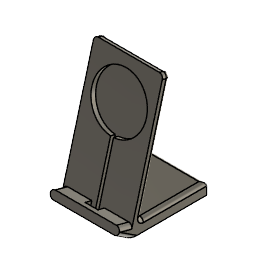
Phone stand (Autodesk Fusion 360 design; units mm, degrees)
part number: 2026-01-15-00-13-54-306
Autodesk Fusion 360 part; units mm, degrees
sketch "Sketch1" plane through (0, 0, 0) normal (1, 0, 0) x (0, 1, 0)
  line L0 (0, 0) -> (70, 0)
  line L1 (70, 0) -> (70, 12)
  line L2 (70, 12) -> (3.2154, 12)
  line L3 (25.9915, 127.9111) -> (33.7189, 125.8405)
  line L4 (33.7189, 125.8405) -> (0.59, 2.202)
  line L5 (0.59, 2.202) -> (-7.1374, 4.2726)
  line L6 (-7.1374, 4.2726) -> (25.9915, 127.9111)
  line L7 (-7.1374, 4.2726) -> (-19.6944, 7.6372)
  line L8 (-19.6944, 7.6372) -> (-17.6239, 15.3646)
  line L9 (-17.6239, 15.3646) -> (-5.0668, 12)
  line L10 (0, 0) -> (3.2154, 12)
  line L11 (-19.6944, 7.6372) -> (-8, 0)
  line L12 (-8, 0) -> (0, 0)
  dimension "d1" = 12
  dimension "d3" = 128
  dimension "d4" = 8
  dimension "d5" = 13
  dimension "d6" = 8
  dimension "d7" = 75
  dimension "d8" = 70
  dimension "d10" = 12
  dimension "d11" = 8
  constraint horizontal L0
  constraint vertical L1
  constraint horizontal L2
  constraint coincident L0.start L10.start
  constraint perpendicular L6 L7
  constraint perpendicular L7 L8
  constraint coincident L6 L9.end
  constraint perpendicular L6 L9
  constraint parallel L4 L10
  constraint coincident L4 L2.end
  constraint perpendicular L4 L5
  constraint perpendicular L1 L12
  measures "d1" distance of L0 L2
  measures "d3" distance of L3 L5
  measures "d4" distance of L4 L6
  measures "d5" distance of L6 L8
  measures "d6" distance of L7 L9
  measures "d7" angle of L2 L4
  measures "d8" distance of L0.start L1
  measures "d10" distance of L9.end L12
  measures "d11" distance of L0.start L11.end
extrude "Extrude1" add sketch "Sketch1" along normal blind 70
sketch "Sketch2" plane through (0, -7.7274, 2.0706) normal (0, -0.965926, 0.258819) x (1, 0, 0)
  line L0 (0, 130.2797) -> (0, 10.2797)
  line L1 (0, 10.2797) -> (70, 10.2797)
  line L2 (70, 10.2797) -> (70, 130.2797)
  line L3 (70, 130.2797) -> (0, 130.2797)
  circle A0 centre (35, 92.2797) radius 27.75
  line L4 (33.5, 10.2797) -> (36.5, 10.2797)
  line L5 (36.5, 10.2797) -> (36.5, 64.5703)
  line L6 (33.5, 64.5703) -> (33.5, 10.2797)
  dimension "d14" = 55.5
  dimension "d15" = 82
  dimension "d16" = 35
  dimension "d17" = 3
  constraint horizontal L4
  constraint vertical L5
  constraint vertical L6
  constraint coincident L1 L4.start
  constraint coincident A0 L6.start
  constraint coincident A0 L5.end
  constraint midpoint L1 L4
  measures "d14" diameter of A0
  measures "d15" distance of L1 A0.centre
  measures "d16" distance of L2 A0.centre
  measures "d17" distance of L5 L6
extrude "Extrude2" cut sketch "Sketch2" against normal blind 5 contours L1 A0 L4 L5 L6 | A0
sketch "Sketch3" plane through (0, 2.6606, 9.9294) normal (0, 0.258819, 0.965926) x (-1, 0, 0)
  line L0 (0, 8) -> (0, 21)
  line L1 (0, 21) -> (-70, 21)
  line L2 (-70, 21) -> (-70, 8)
  line L3 (-70, 8) -> (-36.5, 8)
  line L4 (-36.5, 8) -> (-36.5, 3)
  line L5 (-36.5, 3) -> (-33.5, 3)
  line L6 (-33.5, 3) -> (-33.5, 8)
  line L7 (-33.5, 8) -> (0, 8)
  line L8 (-28.5, 8) -> (-41.5, 8)
  line L9 (-41.5, 8) -> (-41.5, 15)
  line L10 (-41.5, 15) -> (-28.5, 15)
  line L11 (-28.5, 15) -> (-28.5, 8)
  line L12 (-33.5, 3) -> (-36.5, 3)
  line L13 (-36.5, 3) -> (-36.5, 8)
  line L14 (-36.5, 8) -> (-33.5, 8)
  line L15 (-33.5, 8) -> (-33.5, 3)
  dimension "d20" = 13
  dimension "d21" = 7
  constraint horizontal L8
  constraint vertical L9
  constraint horizontal L10
  constraint vertical L11
  constraint collinear L3 L8
  constraint horizontal L12
  constraint vertical L13
  constraint horizontal L14
  constraint vertical L15
  constraint coincident L3.end L4.start
  constraint coincident L5.end L6.start
  constraint midpoint L8 L14
  measures "d20" distance of L9 L11
  measures "d21" distance of L8 L10
extrude "Extrude3" cut sketch "Sketch3" against normal blind 13 contours L3 L7 L8 L9 L10 L11 L14 | L4 L5 L6 L8 L12 L13 L14 L15
sketch "Sketch4" plane through (0, 0, 0) normal (0, 0, -1) x (1, 0, 0)
  line L0 (33.5, 3.1058) -> (33.5, 8)
  line L1 (33.5, 8) -> (0, 8)
  line L2 (0, 8) -> (0, -70)
  line L3 (0, -70) -> (70, -70)
  line L4 (70, -70) -> (70, 8)
  line L5 (70, 8) -> (36.5, 8)
  line L6 (36.5, 8) -> (36.5, 3.1058)
  line L7 (36.5, 3.1058) -> (33.5, 3.1058)
  line L8 (33.5, 3.1058) -> (36.5, 3.1058)
  line L9 (36.5, 3.1058) -> (36.5, -70)
  line L10 (36.5, -70) -> (33.5, -70)
  line L11 (33.5, -70) -> (33.5, 3.1058)
  circle A0 centre (35, -31) radius 25
  dimension "d24" = 3
  dimension "d25" = 39
  dimension "d26" = 35
  dimension "d27" = 50
  constraint horizontal L8
  constraint vertical L9
  constraint horizontal L10
  constraint vertical L11
  constraint coincident L3 L9.end
  constraint coincident L0.start L7.end
  measures "d24" distance of L9 L11
  measures "d25" distance of L3 A0.centre
  measures "d26" distance of L4 A0.centre
  measures "d27" diameter of A0
extrude "Extrude4" cut sketch "Sketch4" against normal blind 3.5 contours L7 L8 L9 L11 A0 | L9 L11 A0 | L3 L9 L10 L11 A0
fillet "Fillet2" radius 4 4 edges at (0, -11.3453, 13.6823) (0, -13.8472, 3.8186) (70, -11.3453, 13.6823) (70, -13.8472, 3.8186)
fillet "Fillet3" radius 2 1 edges at (35, 3.2154, 12)
fillet "Fillet4" radius 4 7 edges at (70, 37.9109, 12) (70, 4.2351, 12.7825) (70, 18.8044, 70.1791) (0, 37.9109, 12) (0, 4.2351, 12.7825) (0, 18.8044, 70.1791) (35, 70, 12)
fillet "Fillet5" radius 4 5 edges at (0, 27.9233, 127.3935) (1.1716, 32.5872, 126.1438) (35, 33.7189, 125.8405) (68.8284, 32.5872, 126.1438) (70, 27.9233, 127.3935)
fillet "Fillet6" radius 6 1 edges at (35, -2.168, 3.5)
sketch "Sketch5" plane through (0, 0, 3.5) normal (0, 0, -1) x (1, 0, 0)
  line L0 (36.5, -5.6513) -> (33.5, -5.6513)
  line L1 (33.5, -5.6513) -> (33.5, -70)
  line L2 (33.5, -70) -> (36.5, -70)
  line L3 (36.5, -70) -> (36.5, -5.6513)
  line L4 (33.5, -6) -> (34, -6)
  line L5 (34, -6) -> (34, -6.5)
  line L6 (34, -6.5) -> (33.5, -6.5)
  line L7 (33.5, -6.5) -> (33.5, -6)
  line L8 (36.5, -6) -> (36, -6)
  line L9 (36, -6) -> (36, -6.5)
  line L10 (36, -6.5) -> (36.5, -6.5)
  line L11 (36.5, -6.5) -> (36.5, -6)
  line L12 (33.5, -57.5) -> (34, -57.5)
  line L13 (34, -57.5) -> (34, -58)
  line L14 (34, -58) -> (33.5, -58)
  line L15 (33.5, -58) -> (33.5, -57.5)
  line L16 (36.5, -57.5) -> (36, -57.5)
  line L17 (36, -57.5) -> (36, -58)
  line L18 (36, -58) -> (36.5, -58)
  line L19 (36.5, -58) -> (36.5, -57.5)
  dimension "d44" = 0.5
  dimension "d45" = 0.5
  dimension "d46" = 0.5
  dimension "d47" = 0.5
  dimension "d51" = 0.5
  dimension "d52" = 0.5
  dimension "d53" = 0.5
  dimension "d54" = 0.5
  dimension "d55" = 12
  constraint horizontal L4
  constraint vertical L5
  constraint horizontal L6
  constraint vertical L7
  constraint coincident L1 L4.start
  constraint horizontal L8
  constraint vertical L9
  constraint horizontal L10
  constraint vertical L11
  constraint coincident L3 L8.start
  constraint collinear L4 L8
  constraint horizontal L12
  constraint vertical L13
  constraint horizontal L14
  constraint vertical L15
  constraint coincident L1 L12.start
  constraint horizontal L16
  constraint vertical L17
  constraint horizontal L18
  constraint vertical L19
  constraint coincident L3 L16.start
  constraint collinear L12 L16
  measures "d44" distance of L5 L7
  measures "d45" distance of L4 L6
  measures "d46" distance of L8.start L8.end
  measures "d47" distance of L8 L10
  measures "d51" distance of L12 L14
  measures "d52" distance of L13 L15
  measures "d53" distance of L16 L18
  measures "d54" distance of L17 L19
  measures "d55" distance of L2 L14
extrude "Extrude6" add sketch "Sketch5" along normal blind 3.5 contours L3 L8 L9 L10 L11 | L1 L4 L5 L6 L7 | L3 L16 L17 L18 L19 | L1 L12 L13 L14 L15
equation "d25 = ( 78 / 2 ) * 1 mm"
